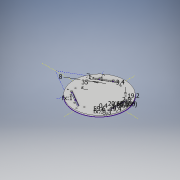
# Autodesk Inventor part: Stewart-Platform-Base-Innenanordnung
Saved by Autodesk Inventor 2018.2 (Build 222227000, 227)
## iProperties
Created: 2018-02-17
Part Number: Stewart-Platform-Base-Innenanordnung
Material: Generisch
Document SubType Name: Modeling
Designer: JochenAlt
Density: 1 g/cm^3
Appearance: Vorgabe
Author: JochenAlt
Autodesk Inventor part; units mm, degrees
ref_plane "YZ Plane" through (0, 0, 0) normal (1, 0, 0) x (0, 1, 0)
ref_plane "XZ Plane" through (0, 0, 0) normal (0, 1, 0) x (-1, 0, 0)
ref_plane "XY Plane" through (0, 0, 0) normal (0, 0, 1) x (1, 0, 0)
sketch "Skizze1" plane through (0, 0, 0) normal (0, 0, 1) x (1, 0, 0)
  line L0 (0, 78.781) -> (0, -78.781) construction
  line L1 (-128.8214, 0) -> (87.1211, 0) construction
  line L2 (31.7862, 29.8) -> (44.1862, 29.8) construction
  line L3 (47.5862, 26.4) -> (47.5862, -26.4) construction
  line L4 (44.1862, -29.8) -> (31.7862, -29.8) construction
  line L5 (28.3862, -26.4) -> (28.3862, 26.4) construction
  arc A0 (31.7862, 29.8) -> (28.3862, 26.4) centre (31.7862, 26.4) ccw construction
  arc A1 (47.5862, 26.4) -> (44.1862, 29.8) centre (44.1862, 26.4) ccw construction
  arc A2 (44.1862, -29.8) -> (47.5862, -26.4) centre (44.1862, -26.4) ccw construction
  arc A3 (28.3862, -26.4) -> (31.7862, -29.8) centre (31.7862, -26.4) ccw construction
  circle A4 centre (31.7862, 26.4) radius 1.4
  circle A5 centre (44.1862, 26.4) radius 1.4
  circle A6 centre (31.7862, -26.4) radius 1.4
  circle A7 centre (44.1862, -26.4) radius 1.4
  line L6 (41.6862, 21.4) -> (41.6862, -21.4)
  line L7 (38.3862, 21.4) -> (38.3862, -21.4)
  line L8 (38.3862, 21.4) -> (41.6862, 21.4)
  line L9 (38.3862, -21.4) -> (41.6862, -21.4)
  line L10 (38.3862, 0.8) -> (41.6862, 0.8)
  line L11 (38.3862, -0.8) -> (41.6862, -0.8)
  line L12 (41.6862, 12.5) -> (44.6022, 12.5)
  line L13 (44.6022, 12.5) -> (44.6022, 9.7)
  line L14 (44.6022, 9.7) -> (41.6862, 9.7)
  line L15 (41.6862, -9.7) -> (44.6022, -9.7)
  line L16 (44.6022, -9.7) -> (44.6022, -12.5)
  line L17 (44.6022, -12.5) -> (41.6862, -12.5)
  line L18 (44.1862, 30.2) -> (31.7862, 30.2)
  arc A8 (31.7862, 30.2) -> (27.9862, 26.4) centre (31.7862, 26.4) ccw
  line L19 (27.9862, 26.4) -> (27.9862, -26.4)
  arc A9 (27.9862, -26.4) -> (31.7862, -30.2) centre (31.7862, -26.4) ccw
  line L20 (31.7862, -30.2) -> (44.1862, -30.2)
  arc A10 (44.1862, -30.2) -> (47.9862, -26.4) centre (44.1862, -26.4) ccw
  line L21 (47.9862, -26.4) -> (47.9862, 26.4)
  arc A11 (47.9862, 26.4) -> (44.1862, 30.2) centre (44.1862, 26.4) ccw
  line L22 (25.9381, -29.8698) -> (28.5182, -28.339) construction
  line L23 (-0.6602, 43.9435) -> (-2.3102, 46.8013)
  circle A12 centre (0.77, 51.4664) radius 1.4
  arc A13 (3.7144, 53.1664) -> (-0.93, 54.4109) centre (0.77, 51.4664) ccw construction
  arc A14 (4.0608, 53.3664) -> (-1.13, 54.7573) centre (0.77, 51.4664) ccw
  circle A15 centre (6.97, 40.7277) radius 1.4
  line L24 (12.899, 37.398) -> (10.2832, 38.867) construction
  arc A16 (8.67, 37.7832) -> (9.9144, 42.4277) centre (6.97, 40.7277) ccw construction
  arc A17 (8.87, 37.4368) -> (10.2608, 42.6277) centre (6.97, 40.7277) ccw
  line L25 (10.2608, 42.6277) -> (4.0608, 53.3664)
  line L26 (3.7144, 53.1664) -> (9.9144, 42.4277) construction
  line L27 (-41.7007, 12.6277) -> (-47.9007, 23.3664) construction
  arc A18 (-41.7007, 12.6277) -> (-37.0562, 11.3832) centre (-38.7562, 14.3277) ccw construction
  circle A19 centre (-38.7562, 14.3277) radius 1.4
  circle A20 centre (-44.9562, 25.0664) radius 1.4
  arc A21 (-42.0471, 12.4277) -> (-36.8562, 11.0368) centre (-38.7562, 14.3277) ccw
  line L28 (-48.2471, 23.1664) -> (-42.0471, 12.4277)
  arc A22 (-46.6562, 28.0109) -> (-47.9007, 23.3664) centre (-44.9562, 25.0664) ccw construction
  arc A23 (-46.8562, 28.3573) -> (-48.2471, 23.1664) centre (-44.9562, 25.0664) ccw
  line L29 (-11.4758, 44.8767) -> (-10.0178, 42.3513)
  line L30 (-13.9007, 43.4767) -> (-11.4758, 44.8767)
  line L31 (-12.4427, 40.9513) -> (-13.9007, 43.4767)
  line L32 (-37.7261, 22.5435) -> (-39.3761, 25.4013)
  line L33 (-31.6684, 29.8513) -> (-33.1264, 32.3767)
  line L34 (-33.1264, 32.3767) -> (-30.7016, 33.7767)
  line L35 (-30.7016, 33.7767) -> (-29.2436, 31.2513)
  line L36 (-19.8859, 32.8435) -> (-21.5359, 35.7013)
  line L37 (-18.5003, 33.6435) -> (-20.1503, 36.5013)
  line L38 (-39.3761, 25.4013) -> (-2.3102, 46.8013)
  line L39 (-1.13, 54.7573) -> (-46.8562, 28.3573)
  line L40 (-46.6562, 28.0109) -> (-0.93, 54.4109) construction
  line L41 (8.67, 37.7832) -> (-37.0562, 11.3832) construction
  line L42 (-36.8562, 11.0368) -> (8.87, 37.4368)
  line L43 (-37.7261, 22.5435) -> (-0.6602, 43.9435)
  line L44 (-37.7261, -22.5435) -> (-39.3761, -25.4013)
  circle A24 centre (-44.9562, -25.0664) radius 1.4
  arc A25 (-47.9007, -23.3664) -> (-46.6562, -28.0109) centre (-44.9562, -25.0664) ccw construction
  arc A26 (-48.2471, -23.1664) -> (-46.8562, -28.3573) centre (-44.9562, -25.0664) ccw
  circle A27 centre (-38.7562, -14.3277) radius 1.4
  line L45 (-38.8371, -7.5282) -> (-38.8014, -10.528) construction
  arc A28 (-37.0562, -11.3832) -> (-41.7007, -12.6277) centre (-38.7562, -14.3277) ccw construction
  arc A29 (-36.8562, -11.0368) -> (-42.0471, -12.4277) centre (-38.7562, -14.3277) ccw
  line L46 (-42.0471, -12.4277) -> (-48.2471, -23.1664)
  line L47 (-47.9007, -23.3664) -> (-41.7007, -12.6277) construction
  line L48 (9.9144, -42.4277) -> (3.7144, -53.1664) construction
  arc A30 (9.9144, -42.4277) -> (8.67, -37.7832) centre (6.97, -40.7277) ccw construction
  circle A31 centre (6.97, -40.7277) radius 1.4
  circle A32 centre (0.77, -51.4664) radius 1.4
  arc A33 (10.2608, -42.6277) -> (8.87, -37.4368) centre (6.97, -40.7277) ccw
  line L49 (4.0608, -53.3664) -> (10.2608, -42.6277)
  arc A34 (-0.93, -54.4109) -> (3.7144, -53.1664) centre (0.77, -51.4664) ccw construction
  arc A35 (-1.13, -54.7573) -> (4.0608, -53.3664) centre (0.77, -51.4664) ccw
  line L50 (-33.1264, -32.3767) -> (-31.6684, -29.8513)
  line L51 (-30.7016, -33.7767) -> (-33.1264, -32.3767)
  line L52 (-29.2436, -31.2513) -> (-30.7016, -33.7767)
  line L53 (-0.6602, -43.9435) -> (-2.3102, -46.8013)
  line L54 (-10.0178, -42.3513) -> (-11.4758, -44.8767)
  line L55 (-11.4758, -44.8767) -> (-13.9007, -43.4767)
  line L56 (-13.9007, -43.4767) -> (-12.4427, -40.9513)
  line L57 (-18.5003, -33.6435) -> (-20.1503, -36.5013)
  line L58 (-19.8859, -32.8435) -> (-21.5359, -35.7013)
  line L59 (-2.3102, -46.8013) -> (-39.3761, -25.4013)
  line L60 (-46.8562, -28.3573) -> (-1.13, -54.7573)
  line L61 (-0.93, -54.4109) -> (-46.6562, -28.0109) construction
  line L62 (-37.0562, -11.3832) -> (8.67, -37.7832) construction
  line L63 (8.87, -37.4368) -> (-36.8562, -11.0368)
  line L64 (-0.6602, -43.9435) -> (-37.7261, -22.5435)
  line L65 (-31.914, 33.0767) -> (-43.6029, 53.3224) construction
  line L66 (-34.106, 36.8733) -> (-97.9725, 0) construction
  line L67 (-31.914, -33.0767) -> (-43.7977, -53.6598) construction
  line L68 (-34.106, -36.8733) -> (-97.9725, 0) construction
  circle A36 centre (0, 0) radius 56.2722
  line L69 (-49.1485, 27.404) -> (-48.2751, 26.917) construction
  line L70 (-42.6725, 30.3109) -> (-25.1725, 0) construction
  dimension "d1" = 59.6
  dimension "d2" = 19.2
  dimension "d3" = 3.4
  dimension "d5" = 2.8
  dimension "d6" = 5.9
  dimension "d7" = 3.3
  dimension "d8" = 20.6
  dimension "d9" = 1.6
  dimension "d10" = 2.984
  dimension "d11" = 2.8
  dimension "d12" = 19.4
  dimension "d21" = 0.4
  dimension "d22" = 3
  dimension "d32" = 360
  dimension "d44" = 1
  dimension "d45" = 1
  dimension "d47" = 1
  dimension "d53" = 35
  dimension "d54" = 8
  constraints: 138 end point, 52 point on circle, 36 centre point, 30 point on line, 13 coincident, 10 perpendicular, 8 tangent, 6 equal radius, 6 horizontal, 6 parallel, 2 line through centre, 2 midpoint, 2 vertical, 1 collinear, 242 other
  measures "d1" distance between parallel lines of L4 L2
  measures "d2" distance between parallel lines of L3 L5
  measures "d3" radius of A0
  measures "d5" diameter of A4
  measures "d6" distance between parallel lines of L3 L6
  measures "d7" distance between parallel lines of L6 L7
  measures "d8" distance between parallel lines of L10 L8
  measures "d9" distance between parallel lines of L11 L10
  measures "d10" distance between parallel lines of L3 L13
  measures "d11" distance between parallel lines of L14 L12
  measures "d12" distance between parallel lines of L15 L14
  measures "d21" distance between parallel lines of L19 L5
  measures "d22" distance of L22.end L22.start
  measures "d44" distance between parallel lines of L39 L66
  measures "d45" distance between parallel lines of L68 L60
  measures "d47" distance of L69.start L69.end
  measures "d53" distance of L70.start L70.end
  measures "d54" distance between parallel lines of L70 L27
extrude "Extrusion5" add sketch "Skizze1" along normal blind 3 contours A11 L21 A10 L20 A9 L19 A8 L18 | L25 A17 L42 A21 L28 A23 L39 A14 | L46 A29 L63 A33 L49 A35 L60 A26 | A36
extrude "Extrusion4" cut sketch "Skizze1" along normal blind 1 contours L10 L6 L11 L7 | A11 L21 A10 L20 A9 L19 A8 L18 | L43 L36 L38 L37 | L25 A17 L42 A21 L28 A23 L39 A14 | L64 L57 L59 L58 | L46 A29 L63 A33 L49 A35 L60 A26
equation "\"d22\" = d20"
equation "\"d20\" = 3"
